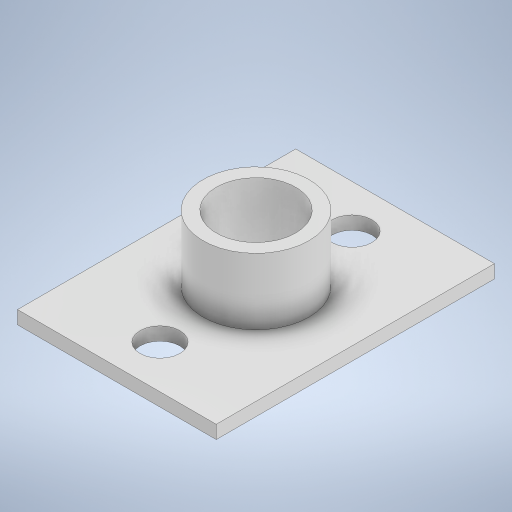
# Autodesk Inventor part: bearing_shaft_base_mount
Saved by Autodesk Inventor 2024 (Build 280153000, 153)
## iProperties
Created: 2025-12-10
Part Number: bearing_shaft_base_mount
Material: PET Plastic
Document SubType Name: Modeling
Designer: schar
Density: 1.541 g/cm^3
Appearance: Polycarbonate - Clear
Author: schar
Autodesk Inventor part; units mm, degrees
ref_plane "YZ Plane" through (0, 0, 0) normal (1, 0, 0) x (0, 1, 0)
ref_plane "XZ Plane" through (0, 0, 0) normal (0, 1, 0) x (-1, 0, 0)
ref_plane "XY Plane" through (0, 0, 0) normal (0, 0, 1) x (1, 0, 0)
sketch "Sketch1" plane through (0, 0, 0) normal (0, 1, 0) x (-1, 0, 0)
  line L0 (0, 0) -> (30, 0)
  line L1 (30, 0) -> (30, -42)
  line L2 (30, -42) -> (0, -42)
  line L3 (0, -42) -> (0, 0)
  line L4 (0, 0) -> (15, 0)
  line L5 (15, 0) -> (15, -6.5)
  circle A0 centre (15, -6.5) radius 3
  line L6 (15, -42) -> (15, -35.5)
  circle A1 centre (15, -35.5) radius 3
  line L7 (5, -21) -> (15, -21)
  circle A2 centre (15, -21) radius 6
  circle A3 centre (15, -21) radius 8
  line L8 (15, 0) -> (15, -21)
  dimension "d0" = 30
  dimension "d1" = 42
  dimension "d2" = 15
  dimension "d3" = 6.5
  dimension "d5" = 6
  dimension "d6" = 6.5
  dimension "d7" = 6
  dimension "d8" = 12
  dimension "d10" = 21
  constraints: 18 end point, 4 centre point, 4 coincident, 3 perpendicular, 2 horizontal, 2 midpoint, 2 parallel, 1 vertical
  measures "d0" distance of L1.end L2.end
  measures "d1" distance of L0.end L1.end
  measures "d2" distance of L0.start L4.end
  measures "d3" distance of L4.end L5.end
  measures "d5" diameter of A0
  measures "d6" distance of L6.start L6.end
  measures "d7" diameter of A1
  measures "d8" diameter of A2
  measures "d10" distance of L4.end L7.end
extrude "Extrusion1" add sketch "Sketch1" along normal blind 2 contours A3 L7 A2 L8 | L8 A2 L7 A3 | L0 L1 L2 L3
sketch "Sketch2" plane through (0, 2, 0) normal (0, 1, 0) x (1, 0, 0)
  line L0 (-30, 0) -> (0, 0) projected
  line L1 (-15, 0) -> (-15, 21)
  circle A0 centre (-15, 21) radius 6 projected
  circle A1 centre (-15, 21) radius 8
  circle A2 centre (-15, 21) radius 6
  dimension "d13" = 21
  constraints: 2 centre point, 2 coincident, 2 end point, 1 concentric, 1 midpoint, 1 vertical
  measures "d13" distance of L1.start L1.end
extrude "Extrusion2" add sketch "Sketch2" along normal blind 10
body "Solid1"
